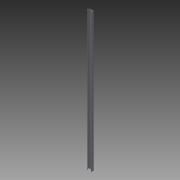
# Autodesk Inventor part: 2in rail
Saved by Autodesk Inventor 2015 SP1 (Build 190203100, 203)
## iProperties
Created: 2015-01-11
Part Number: 2in rail
Material: Generic
Document SubType Name: Modeling
Designer: Jarod
Density: 1 g/cm^3
Appearance: Default
Author: Jarod
Autodesk Inventor part; units mm, degrees
ref_plane "YZ Plane" through (0, 0, 0) normal (1, 0, 0) x (0, 1, 0)
ref_plane "XZ Plane" through (0, 0, 0) normal (0, 1, 0) x (-1, 0, 0)
ref_plane "XY Plane" through (0, 0, 0) normal (0, 0, 1) x (1, 0, 0)
sketch "Sketch1" plane through (0, 0, 0) normal (0, 1, 0) x (-1, 0, 0)
  line L0 (0, 0) -> (50.8, 0) construction
  line L1 (50.8, 0) -> (50.8, -12.7) construction
  line L2 (50.8, -12.7) -> (0, -12.7) construction
  line L3 (0, -12.7) -> (0, 0) construction
  line L4 (50.8, -12.7) -> (50.8, -25.4) construction
  line L5 (50.8, -12.7) -> (63.5, -12.7) construction
  line L6 (33.4515, -25.4) -> (0, -25.4) construction
  line L7 (0, -25.4) -> (0, -12.7) construction
  circle A0 centre (44.45, -12.7) radius 6.35 construction
  circle A1 centre (6.35, -12.7) radius 6.35 construction
  arc A2 (50.8, -12.7) -> (47.625, -7.2007) centre (44.45, -12.7) ccw construction
  line L8 (50.8, -12.7) -> (44.45, -12.7) construction
  line L9 (47.625, -7.2007) -> (44.45, -12.7) construction
  arc A3 (47.625, -18.1993) -> (50.8, -12.7) centre (44.45, -12.7) ccw construction
  line L10 (50.8, -12.7) -> (44.45, -12.7) construction
  line L11 (47.625, -18.1993) -> (44.45, -12.7) construction
  line L12 (47.625, -7.2007) -> (35.8129, -0.381) construction
  line L13 (47.625, -7.2007) -> (61.2645, -7.2007) construction
  line L14 (47.625, -18.1993) -> (36.6265, -24.5493) construction
  line L15 (47.625, -18.1993) -> (60.325, -18.1993) construction
  line L16 (35.153, -25.4) -> (0, -25.4) construction
  line L17 (0, -25.4) -> (0, 0) construction
  arc A4 (33.4515, -25.4) -> (36.6265, -24.5493) centre (33.4515, -19.05) ccw construction
  line L18 (0, 0) -> (-1.5875, 0) construction
  line L19 (-1.5875, 0) -> (-1.5875, -26.9875) construction
  line L20 (37.0518, -26.1368) -> (48.4188, -19.5741) construction
  line L21 (-1.5875, -26.9875) -> (33.8768, -26.9875) construction
  arc A5 (33.8768, -26.9875) -> (37.0518, -26.1368) centre (33.8768, -20.6375) ccw construction
  line L22 (36.6066, 0.9938) -> (48.4188, -5.8259) construction
  line L23 (35.534, 0.6599) -> (35.5657, 0.7149) construction
  arc A6 (35.534, 0.6599) -> (35.8129, -0.381) centre (36.1939, 0.2789) ccw construction
  arc A7 (36.6066, 0.9938) -> (35.5657, 0.7149) centre (36.2256, 0.3339) ccw construction
  arc A8 (48.4188, -19.5741) -> (48.4188, -5.8259) centre (44.45, -12.7) ccw construction
  line L24 (0, 0) -> (-1.5875, 0)
  line L25 (-1.5875, 0) -> (-1.5875, -26.9875)
  line L26 (-1.5875, -26.9875) -> (33.8768, -26.9875)
  arc A9 (33.8768, -26.9875) -> (37.0518, -26.1368) centre (33.8768, -20.6375) ccw
  line L27 (37.0518, -26.1368) -> (48.4188, -19.5741)
  arc A10 (48.4188, -19.5741) -> (48.4188, -5.8259) centre (44.45, -12.7) ccw
  line L28 (48.4188, -5.8259) -> (36.6066, 0.9938)
  arc A11 (36.6066, 0.9938) -> (35.8129, -0.381) centre (36.2097, 0.3064) ccw
  line L29 (35.8129, -0.381) -> (47.625, -7.2007)
  arc A12 (47.625, -18.1993) -> (47.625, -7.2007) centre (44.45, -12.7) ccw
  line L30 (47.625, -18.1993) -> (36.6265, -24.5493)
  arc A13 (33.4515, -25.4) -> (36.6265, -24.5493) centre (33.4515, -19.05) ccw
  line L31 (33.4515, -25.4) -> (0, -25.4)
  line L32 (0, -25.4) -> (0, 0)
  point P0 (35.153, 0)
  dimension "d0" = 50.8
  dimension "d1" = 12.7
  dimension "d2" = 12.7
  dimension "d3" = 90
  dimension "d4" = 50.8
  dimension "d5" = 90
  dimension "d6" = 12.7
  dimension "d7" = 12.7
  dimension "d8" = 6.35
  dimension "d9" = 6.35
  dimension "d10" = 6.35
  dimension "d11" = 60
  dimension "d12" = 6.35
  dimension "d13" = 60
  dimension "d14" = 150
  dimension "d15" = 150
  dimension "d16" = 6.35
  dimension "d17" = 1.5875
  dimension "d18" = 26.9875
  dimension "d19" = 90
  dimension "d23" = 1.5875
  dimension "d24" = 90
  dimension "d25" = 6.35
  dimension "d26" = 1.5875
  dimension "d27" = 90
  dimension "d28" = 0.762
  dimension "d29" = 1.5875
  dimension "d30" = 0.7937
  constraints: 66 end point, 24 point on circle, 21 tangent, 14 centre point, 8 point on line, 6 horizontal, 5 collinear, 3 equal length, 3 perpendicular, 2 equal radius, 2 parallel, 1 vertical
  measures "d0" distance of L1.end L2.end
  measures "d1" distance of L0.end L1.end
  measures "d2" distance of L1.end L4.end
  measures "d3" angle of L4 L5
  measures "d4" distance of L4.end L6.end
  measures "d5" angle of L4 L6
  measures "d6" diameter of A0
  measures "d7" diameter of A1
  measures "d8" distance from line of L1 A0.centre
  measures "d9" distance from line of L3 A1.centre
  measures "d10" radius of A2
  measures "d11" angle of L8 L9
  measures "d12" radius of A3
  measures "d13" angle of L11 L10
  measures "d14" angle of L13 L12
  measures "d15" angle of L14 L15
  measures "d16" radius of A4
  measures "d17" distance of L0.start L18.end
  measures "d18" distance of L18.end L19.end
  measures "d19" angle of L19 L18
  measures "d23" distance between parallel lines of L14 L20
  measures "d24" angle of L19 L21
  measures "d25" radius of A5
  measures "d26" distance between parallel lines of L22 L12
  measures "d27" angle of L23 L12
  measures "d28" radius of A6
  measures "d29" radial gap between concentric circles of A2 A8
  measures "d30" radius of A11
extrude "Extrusion1" add sketch "Sketch1" along normal blind 1524
body "Solid1"
